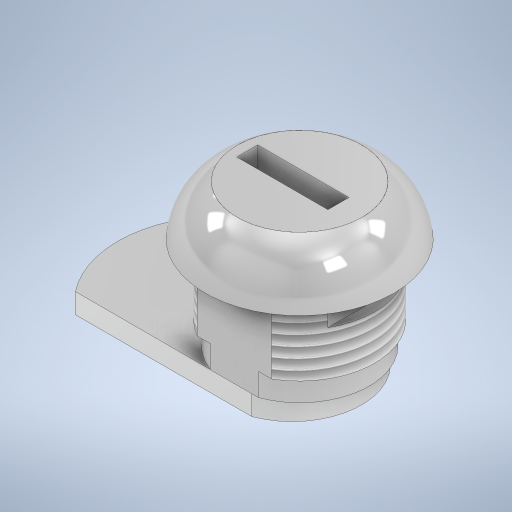
# Autodesk Inventor part: KeyLock
Saved by Autodesk Inventor 2024 (Build 280153000, 153)
## iProperties
Created: 2023-06-10
Part Number: KeyLock
Material: Generic
Document SubType Name: Modeling
Designer: 18179
Density: 1 g/cm^3
Appearance: Aluminum - Dark
Author: 18179
Autodesk Inventor part; units mm, degrees
ref_plane "YZ Plane" through (0, 0, 0) normal (1, 0, 0) x (0, 1, 0)
ref_plane "XZ Plane" through (0, 0, 0) normal (0, 1, 0) x (-1, 0, 0)
sketch "Sketch1" plane through (0, 0, 0) normal (0, 1, 0) x (-1, 0, 0)
  line L0 (0, 0) -> (0, -16.05)
  circle A0 centre (0, -8.025) radius 9.2329
  line L1 (0, 0) -> (4.5657, 0)
  line L2 (0, 0) -> (-4.5657, 0)
  line L3 (0, -16.05) -> (4.5657, -16.05)
  line L4 (0, -16.05) -> (-4.5657, -16.05)
  line L5 (0, -8.025) -> (8.0264, -8.025)
  line L6 (8.0264, -8.025) -> (-8.0264, -8.025)
  line L7 (-8.0264, -8.025) -> (-8.0264, -3.4617)
  line L8 (-8.0264, -8.025) -> (-8.0264, -12.5883)
  line L9 (8.0264, -8.025) -> (8.0264, -12.5883)
  line L10 (8.0264, -8.025) -> (8.0264, -3.4617)
  dimension "d1" = 18.4658
  dimension "d0" = 16.05
  dimension "d2" = 8.0264
  dimension "d3" = 16.0528
  constraints: 22 end point, 5 point on line, 2 horizontal, 2 parallel, 1 midpoint, 1 perpendicular, 1 vertical, 10 other
  measures "d0" distance of L0.start L0.end
  measures "d2" distance of L5.start L5.end
  measures "d3" distance of L5.end L6.end
extrude "Extrusion1" add sketch "Sketch1" along normal blind 3.2004 contours L1 A0 L10 L5 L0 | L0 L6 L7 A0 L2 | L5 L9 A0 L3 L0 | L0 L4 A0 L8 L6
sketch "Sketch2" plane through (0, 0, 0) normal (0, -1, 0) x (1, 0, 0)
  line L0 (8.0264, -3.4617) -> (8.0264, -12.5883) projected
  arc A0 (8.0264, -3.4617) -> (4.5657, 0) centre (0, -8.025) ccw projected
  line L1 (-4.5657, 0) -> (4.5657, 0) projected
  arc A1 (-4.5657, 0) -> (-8.0264, -3.4617) centre (0, -8.025) ccw projected
  line L2 (-8.0264, -12.5883) -> (-8.0264, -3.4617) projected
  arc A2 (-8.0264, -12.5883) -> (-4.5657, -16.05) centre (0, -8.025) ccw projected
  line L3 (4.5657, -16.05) -> (-4.5657, -16.05) projected
  arc A3 (4.5657, -16.05) -> (8.0264, -12.5883) centre (0, -8.025) ccw projected
  circle A4 centre (0, -8.025) radius 9.2329
  point P0 (0, 0)
  point P1 (-8.0264, -3.4617)
  constraints: 1 coincident, 3 other
extrude "Extrusion2" add sketch "Sketch2" along normal blind 5.461 contours A4 L0 | L0 A3 L3 A2 L2 A1 L1 A0 | L2 A4
thread "Thread1" size "3/4-20 UNEF" class "2A" standard "ANSI Unified Screw Threads" full length
sketch "Sketch3" plane through (0, -5.461, 0) normal (0, -1, 0) x (1, 0, 0)
  arc A0 (4.5657, -16.05) -> (4.5657, 0) centre (0, -8.025) ccw projected
  line L0 (4.5657, 0) -> (-4.5657, 0) projected
  arc A1 (-4.5657, 0) -> (-4.5657, -16.05) centre (0, -8.025) ccw projected
  line L1 (-4.5657, -16.05) -> (4.5657, -16.05) projected
  circle A2 centre (0, -8.025) radius 8.5471
  point P0 (0, 0)
  point P1 (2.9415, 0)
  point P2 (-2.9415, 0)
  point P3 (-2.9415, -16.05)
  point P4 (2.9415, -16.05)
  dimension "d10" = 17.0942
  constraints: 1 centre point, 1 coincident
  measures "d10" diameter of A2
extrude "Extrusion3" add sketch "Sketch3" along normal blind 2.794 contours L1 A2 L0
sketch "Sketch4" plane through (0, -8.255, 0) normal (0, -1, 0) x (1, 0, 0)
  line L0 (2.9415, 0) -> (-2.9415, 0) projected
  arc A0 (-2.9415, 0) -> (-2.9415, -16.05) centre (0, -8.025) ccw projected
  line L1 (-2.9415, -16.05) -> (2.9415, -16.05) projected
  arc A1 (2.9415, -16.05) -> (2.9415, 0) centre (0, -8.025) ccw projected
  line L2 (0, -8.025) -> (0, -15.9625)
  line L3 (0, -15.9625) -> (0, -0.0875)
  line L4 (0, -8.025) -> (7.62, -8.025)
  line L5 (7.62, -8.025) -> (-22.352, -8.025)
  line L6 (7.62, -8.025) -> (-22.352, -8.025)
  line L7 (-22.352, -8.025) -> (-22.352, -15.9081)
  line L8 (-22.352, -15.9081) -> (7.62, -15.9081)
  line L9 (7.62, -15.9081) -> (7.62, -8.025)
  line L10 (7.62, -8.025) -> (-22.352, -8.025)
  line L11 (-22.352, -8.025) -> (-22.352, -0.0365)
  line L12 (-22.352, -0.0365) -> (7.62, -0.0365)
  line L13 (7.62, -0.0365) -> (7.62, -8.025)
  arc A2 (7.62, -8.025) -> (2.1111, -0.0365) centre (-0.9265, -8.025) ccw
  arc A3 (-19.594, -0.0365) -> (-22.352, -8.025) centre (-9.4037, -8.025) ccw
  arc A4 (2.1111, -16.0135) -> (7.62, -8.025) centre (-0.9265, -8.025) ccw
  arc A5 (-22.352, -8.025) -> (-19.594, -16.0135) centre (-9.4037, -8.025) ccw
  point P0 (0, 0)
  point P1 (-19.6757, -15.9081)
  point P2 (2.3748, -15.9081)
  dimension "d13" = 7.9375
  dimension "d14" = 15.875
  dimension "d15" = 7.62
  dimension "d16" = 29.972
  constraints: 24 end point, 8 point on circle, 6 equal length, 4 centre point, 4 point on line, 2 perpendicular, 2 symmetric about line, 2 tangent, 1 horizontal, 1 vertical, 2 other
  measures "d13" distance of L2.start L2.end
  measures "d14" distance of L2.end L3.end
  measures "d15" distance of L2.start L4.end
  measures "d16" distance of L4.end L5.end
extrude "Extrusion4" add sketch "Sketch4" along normal blind 2.4638 contours L12 A2 L4 L5 A0 | A0 L5 A3 L12 | L5 L2 L8 A0 | A0 L8 A5 L5 | A4 L8 L2 L4
sketch "Sketch6" plane through (0, -10.7188, 0) normal (0, -1, 0) x (1, 0, 0)
  line L0 (8.0264, -3.4617) -> (8.0264, -12.5883) projected
  arc A0 (4.5657, -16.05) -> (8.0264, -12.5883) centre (0, -8.025) ccw projected
  line L1 (4.5657, -16.05) -> (-4.5657, -16.05) projected
  arc A1 (-8.0264, -12.5883) -> (-4.5657, -16.05) centre (0, -8.025) ccw projected
  line L2 (-8.0264, -12.5883) -> (-8.0264, -3.4617) projected
  arc A2 (-4.5657, 0) -> (-8.0264, -3.4617) centre (0, -8.025) ccw projected
  line L3 (-4.5657, 0) -> (4.5657, 0) projected
  arc A3 (8.0264, -3.4617) -> (4.5657, 0) centre (0, -8.025) ccw projected
  circle A4 centre (0, -8.025) radius 5.5245
  circle A5 centre (0, -8.025) radius 3.175
  point P0 (0, 0)
  dimension "d19" = 11.049
  dimension "d21" = 6.35
  constraints: 2 centre point, 2 coincident
  measures "d19" diameter of A4
  measures "d21" diameter of A5
extrude "Extrusion5" add sketch "Sketch6" along normal blind 1.27 contours A4
fillet "Fillet1" radius 0.762 2 edges at (-3.175, -11.9888, -8.025) (-5.5245, -11.9888, -8.025)
sketch "Sketch7" plane through (0, 3.2004, 0) normal (0, 1, 0) x (1, 0, 0)
  circle A0 centre (0, 8.025) radius 3.175 projected
  circle A1 centre (0, 8.025) radius 11.6205
  circle A2 centre (0, 8.025) radius 7.6835
  line L0 (-7.6835, 8.025) -> (-6.4487, 8.025)
  line L1 (-6.4487, 8.025) -> (4.7625, 8.025)
  circle A3 centre (0, 8.025) radius 4.7625 projected
  line L2 (4.7625, 8.025) -> (-6.4487, 8.025)
  line L3 (-6.4487, 8.025) -> (-6.4487, 9.3147)
  line L4 (-6.4487, 9.3147) -> (4.7625, 9.3147)
  line L5 (4.7625, 9.3147) -> (4.7625, 8.025)
  line L6 (-6.4487, 8.025) -> (-6.4487, 6.7353)
  line L7 (-6.4487, 6.7353) -> (4.7625, 6.7353)
  line L8 (4.7625, 6.7353) -> (4.7625, 8.025)
  point P0 (0, 0)
  dimension "d25" = 23.241
  dimension "d27" = 3.937
  constraints: 18 end point, 3 equal length, 2 horizontal alignment, 2 symmetric about line, 1 centre point, 1 coincident, 1 horizontal, 1 perpendicular, 1 point on line, 3 other
  measures "d25" diameter of A1
extrude "Extrusion6" add sketch "Sketch7" along normal blind 6.096 contours L4 A0 | A0 L4 A3 | L7 A3 A0 | A0 L7 | A2
ref_plane "Work Plane1" through (-6.4487, 3.2004, -8.0193) normal (0, 0, 1) x (1, 0, 0)
sketch "Sketch8" plane through (-6.4487, 3.2004, -8.0193) normal (0, 0, 1) x (1, 0, 0)
  line L0 (14.1322, 6.096) -> (-1.2348, 6.096) projected
  line L1 (-1.2348, 0) -> (14.1322, 0) projected
  line L2 (6.4487, 0) -> (-5.1718, 0)
  arc A0 (-1.2348, 6.096) -> (-5.1718, 0) centre (2.4894, -0.6285) ccw
  line L3 (6.4487, 0) -> (6.4487, 7.4033)
  line L4 (-1.2348, 6.096) -> (-1.2348, 0)
  point P0 (6.4487, -3.2004)
  dimension "d31" = 11.6205
  constraints: 6 end point, 2 point on circle, 2 vertical, 1 centre point, 1 horizontal, 1 midpoint
  measures "d31" distance of L2.start L2.end
revolve "Revolution1" add sketch "Sketch8" angle 360 about axis through (0, 3.2004, -8.0193) along (0, 1, 0) contours L4 L2 A0
body "Solid1"
